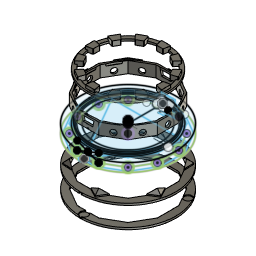
ARC4 v7 (Autodesk Fusion 360 design; units mm, degrees)
Autodesk Fusion 360 part; units mm, degrees
sketch "Sketch1" plane through (0, 0, 0) normal (0, 0, 1) x (1, 0, 0)
  circle A0 centre (0, 0) radius 40
  circle A1 centre (0, 0) radius 39
  circle A2 centre (0, 0) radius 34
  line L0 (0, 0) -> (0, 40)
  circle A3 centre (0, 36.5) radius 2.5
  circle A4 centre (0, 36.5) radius 3.5
  line L1 (3.5, 40) -> (-3.5, 40)
  line L2 (-3.5, 40) -> (-3.5, 33)
  line L3 (-3.5, 33) -> (3.0958, 33)
  line L4 (3.5, 33) -> (3.5, 40)
  line L5 (3.5, 40) -> (-3.5, 33) construction
  line L6 (-3.5, 40) -> (3.5, 33) construction
  line L7 (4.3815, 40) -> (-4.5, 40)
  line L8 (-5, 39.5) -> (-5, 33)
  line L9 (-3.0958, 33) -> (5, 33)
  line L10 (5, 33) -> (5, 40)
  line L11 (5, 40) -> (-5, 33) construction
  line L12 (-5, 40) -> (5, 33) construction
  line L13 (-5, 40) -> (-3.5847, 33.3952)
  line L14 (3.5847, 33.3952) -> (4.8704, 39.3952)
  arc A5 (-4.5, 40) -> (-5, 39.5) centre (-4.5, 39.5) ccw
  arc A6 (4.8704, 39.3952) -> (4.3815, 40) centre (4.3815, 39.5) ccw
  arc A7 (-3.5847, 33.3952) -> (-3.0958, 33) centre (-3.0958, 33.5) ccw
  arc A8 (3.0958, 33) -> (3.5847, 33.3952) centre (3.0958, 33.5) ccw
  line L15 (-10.718, 40) -> (-29.282, 29.282)
  line L16 (-29.282, 29.282) -> (-40, 10.718)
  line L17 (-40, 10.718) -> (-40, -10.718)
  line L18 (-40, -10.718) -> (-29.282, -29.282)
  line L19 (-29.282, -29.282) -> (-10.718, -40)
  line L20 (-10.718, -40) -> (10.718, -40)
  line L21 (10.718, -40) -> (29.282, -29.282)
  line L22 (29.282, -29.282) -> (40, -10.718)
  line L23 (40, -10.718) -> (40, 10.718)
  line L24 (40, 10.718) -> (29.282, 29.282)
  line L25 (29.282, 29.282) -> (10.718, 40)
  line L26 (10.718, 40) -> (-10.718, 40)
  circle A9 centre (0, 0) radius 38
  circle A10 centre (0, 0) radius 42
  line L27 (0, 0) -> (42, 0) construction
  line L28 (-11.2539, 42) -> (-30.7461, 30.7461)
  line L29 (-30.7461, 30.7461) -> (-42, 11.2539)
  line L30 (-42, 11.2539) -> (-42, -11.2539)
  line L31 (-42, -11.2539) -> (-30.7461, -30.7461)
  line L32 (-30.7461, -30.7461) -> (-11.2539, -42)
  line L33 (-11.2539, -42) -> (11.2539, -42)
  line L34 (11.2539, -42) -> (30.7461, -30.7461)
  line L35 (30.7461, -30.7461) -> (42, -11.2539)
  line L36 (42, -11.2539) -> (42, 11.2539)
  line L37 (42, 11.2539) -> (30.7461, 30.7461)
  line L38 (30.7461, 30.7461) -> (11.2539, 42)
  line L39 (11.2539, 42) -> (-11.2539, 42)
  circle A11 centre (0, 0) radius 50
  point P0 (0, 36.5)
  point P1 (0, 36.5)
  dimension "d1" = 80
  dimension "d2" = 78
  dimension "d3" = 68
  dimension "d4" = 7
  dimension "d5" = 7
  dimension "d6" = 10
  dimension "d7" = 7
  dimension "d8" = 0.5
  dimension "d9" = 0.5
  dimension "d19" = 76
  dimension "d20" = 84
  dimension "d37" = 100
  constraint coincident A0.centre A1.centre
  constraint concentric A0 A1
  constraint concentric A0 A2
  constraint coincident A0 L0.end
  constraint vertical L0
  constraint tangent A2 A3
  constraint concentric A3 A4
  constraint coincident L0.end A4
  constraint tangent A0 A4
  constraint horizontal L1
  constraint perpendicular L1 L2
  constraint parallel L1 L3
  constraint parallel L2 L4
  constraint coincident L5 P1
  constraint coincident L6 P1
  constraint coincident P1 P0
  constraint horizontal L7
  constraint perpendicular L7 L8
  constraint parallel L7 L9
  constraint parallel L8 L10
  constraint coincident L11 P1
  constraint coincident L12 P1
  constraint coincident L12.start L7
  constraint coincident L12.start L8
  constraint tangent L7 A5
  constraint tangent L8 A5
  constraint coincident L10.end L7
  constraint coincident L10.end L14
  constraint tangent L7 A6
  constraint tangent L14 A6
  constraint equal A5 A6
  constraint coincident L2.end L13
  constraint coincident L8.end L9
  constraint tangent L13 A7
  constraint tangent L9 A7
  constraint coincident L4.start L14
  constraint coincident L4.start L3
  constraint tangent L14 A8
  constraint tangent L3 A8
  constraint equal A7 A8
  constraint concentric A1 A9
  constraint horizontal L27
  constraint concentric A1 A11
  measures "d1" diameter of A0
  measures "d2" diameter of A1
  measures "d3" diameter of A2
  measures "d4" distance of L2.end L4.start
  measures "d5" distance of L1.end L2.end
  measures "d6" distance of L8.end L9.end
  measures "d7" distance of L12.start L8.end
  measures "d8" radius of A5
  measures "d9" radius of A7
  measures "d19" diameter of A9
  measures "d20" diameter of A10
  measures "d37" diameter of A11
extrude "Extrude1" add sketch "Sketch1" along normal blind 2 contours A0 A1 L8 L10 A5 | A0 L22 L23 | A0 L23 L24 | A0 L24 L25 | A0 L21 L22 | A0 L10 L25 L26 | A0 L20 L21 | A0 A1 L10 L14 A6 | A0 L10 A6 L26 | A0 L19 L20 | A1 L10 L14 A9 | A1 L8 L10 A9 | A0 L18 L19 | A0 L17 L18 | A0 A1 L8 L13 A5 | A1 L8 L13 A9 | A0 L16 L17 | A0 L15 L16 | L13 A5 L26 | A0 L13 A5 L15 L26 | A10 makes body 1
extrude "Extrude2" add sketch "Sketch1" along normal blind 5 separate body contours A0 A1 L4 L14 A6 | A0 L4 L7 A6 L26 | A0 A1 A4 L4 | A0 L1 L4 L7 L26 | A1 L4 L14 A9 | A0 A1 A4 L2 | A1 L0 A4 | A1 L0 A4 | A0 L1 L2 L7 L26 | A1 A4 L4 A9 | A2 L4 L14 A9 | A0 A1 L2 L13 | A0 L2 L7 L13 A5 L26 | A1 A3 A4 A9 | L0 A3 A9 | A1 A3 A4 A9 | L0 A3 A9 | A1 A4 L2 A9 | A4 L4 A9 | A1 L2 L13 A9 | A2 L4 L14 A8 | A0 L13 A5 | L0 A3 A9 | L0 A3 A9 | A2 A3 A4 A9 | A2 A3 A4 A9 | A4 L2 A9 | A2 A4 L4 | A2 L2 L13 A9 | A2 A4 L3 L4 L9 A8 | A2 L0 A4 | A2 L0 A4 | A2 A4 L2 | A2 L2 L13 A7 | A2 A4 L2 L3 L9 A7 makes body 2
pattern_circular "C-Pattern1" count 12 over 360 about axis through (0, 0, 1.75) along (0, 0, 1) of bodies 2 makes body 3 at (-17.1521, 32.7176, 0) makes body 4 at (-31.213, 19.7582, 0) makes body 5 at (-36.9103, 1.5046, 0) makes body 6 at (-32.7176, -17.1521, 0) makes body 7 at (-19.7582, -31.213, 0) makes body 8 at (-1.5046, -36.9103, 0) makes body 9 at (17.1521, -32.7176, 0) makes body 10 at (31.213, -19.7582, 0) makes body 11 at (36.9103, -1.5046, 0) makes body 12 at (32.7176, 17.1521, 0) makes body 13 at (19.7582, 31.213, 0)
combine "Combine1" operation add target body 4 tool bodies 9 2 10 8 13 12 1 11 7 6 3 5
hole "Hole1" at (0, 36.5, 0) direction (0, 0, 1) diameter 3.5 depth 3 tip angle 140 bodies 4
pattern_circular "C-Pattern2" count 12 over 360 about axis through (0, 0, 1.75) along (0, 0, 1) of "Hole1"
extrude "Extrude3" add sketch "Sketch1" against normal blind 9 separate body contours A10 | A10 L35 L36 | A10 L36 L37 | A10 L37 L38 | A10 L34 L35 | A10 L38 L39 | A10 L33 L34 | A10 L28 L39 | A10 L32 L33 | A10 L28 L29 | A10 L31 L32 | A10 L29 L30 | A10 L30 L31 makes body 14
extrude "Extrude4" add sketch "Sketch1" along normal blind 2 from surface at -9 separate body contours A11 makes body 15
sketch "Sketch2" plane through (0, -42, 0) normal (0, -1, 0) x (1, 0, 0)
  line L0 (11.2539, 0) -> (-11.2539, 0)
  line L1 (-11.2539, 0) -> (-11.2539, -9)
  line L2 (-11.2539, -9) -> (11.2539, -9)
  line L3 (11.2539, -9) -> (11.2539, 0)
  line L4 (-11.2539, 0) -> (11.2539, -9)
  line L5 (-11.2539, -9) -> (11.2539, 0)
  circle A0 centre (0, -4.5) radius 2.9
  dimension "d31" = 5.8
  constraint coincident L0.end L1.start
  constraint coincident L2.end L3.start
  constraint coincident L1.end L2.start
  constraint coincident L0.start L3.end
  constraint midpoint L5 A0.centre
  measures "d31" diameter of A0
hole "Hole2" at (0, -42, -4.5) direction (0, 1, 0) diameter 5.8 depth 10 tip angle 140 bodies 14
pattern_circular "C-Pattern3" count 12 over 360 about axis through (0, 0, 1.75) along (0, 0, 1) of "Hole2"
sketch "Sketch4" plane through (0, 0, -9) normal (0, 0, 1) x (1, 0, 0)
  line L0 (-11.2539, 42) -> (11.2539, 42)
  line L1 (-30.7461, 30.7461) -> (-11.2539, 42)
  line L2 (-42, 11.2539) -> (-30.7461, 30.7461)
  line L3 (-42, -11.2539) -> (-42, 11.2539)
  line L4 (-30.7461, -30.7461) -> (-42, -11.2539)
  line L5 (-11.2539, -42) -> (-30.7461, -30.7461)
  line L6 (11.2539, -42) -> (-11.2539, -42)
  line L7 (30.7461, -30.7461) -> (11.2539, -42)
  line L8 (42, -11.2539) -> (30.7461, -30.7461)
  line L9 (42, 11.2539) -> (42, -11.2539)
  line L10 (30.7461, 30.7461) -> (42, 11.2539)
  circle A0 centre (0, 0) radius 50
  line L11 (0, -46) -> (39.8372, 23)
  line L12 (39.8372, 23) -> (-39.8372, 23)
  line L13 (-39.8372, 23) -> (0, -46)
  circle A1 centre (0, -46) radius 4.1
  line L14 (30.7461, 30.7461) -> (11.2539, 42)
  line L15 (11.2539, 42) -> (-11.2539, 42)
  line L16 (-11.2539, 42) -> (-30.7461, 30.7461)
  line L17 (-30.7461, 30.7461) -> (-42, 11.2539)
  line L18 (-42, 11.2539) -> (-42, -11.2539)
  line L19 (-42, -11.2539) -> (-30.7461, -30.7461)
  line L20 (-30.7461, -30.7461) -> (-11.2539, -42)
  line L21 (-11.2539, -42) -> (11.2539, -42)
  line L22 (11.2539, -42) -> (30.7461, -30.7461)
  line L23 (30.7461, -30.7461) -> (42, -11.2539)
  line L24 (42, -11.2539) -> (42, 11.2539)
  line L25 (42, 11.2539) -> (30.7461, 30.7461)
  circle A2 centre (0, 0) radius 50
  line L26 (11.2539, 42) -> (-11.2539, 42)
  line L27 (11.2539, 42) -> (0, 42)
  line L28 (3, 49.1142) -> (-3, 49.1142)
  line L29 (-3, 49.1142) -> (-3, 34.8858)
  line L30 (-3, 34.8858) -> (3, 34.8858)
  line L31 (3, 34.8858) -> (3, 49.1142)
  line L32 (3, 49.1142) -> (-3, 34.8858) construction
  line L33 (-3, 49.1142) -> (3, 34.8858) construction
  line L34 (-12.5936, 47) -> (-34.4064, 34.4064)
  line L35 (-34.4064, 34.4064) -> (-47, 12.5936)
  line L36 (-47, 12.5936) -> (-47, -12.5936)
  line L37 (-47, -12.5936) -> (-34.4064, -34.4064)
  line L38 (-34.4064, -34.4064) -> (-12.5936, -47)
  line L39 (-12.5936, -47) -> (12.5936, -47)
  line L40 (12.5936, -47) -> (34.4064, -34.4064)
  line L41 (34.4064, -34.4064) -> (47, -12.5936)
  line L42 (47, -12.5936) -> (47, 12.5936)
  line L43 (47, 12.5936) -> (34.4064, 34.4064)
  line L44 (34.4064, 34.4064) -> (12.5936, 47)
  line L45 (12.5936, 47) -> (-12.5936, 47)
  line L46 (11.2539, 42) -> (12.5936, 47)
  line L47 (12.5936, 47) -> (3, 42)
  line L48 (12.5936, 47) -> (18.4019, 37.8731)
  line L49 (0, 42) -> (0, 49.1142)
  line L50 (-12.5936, 47) -> (-3, 42)
  line L51 (-12.5936, 47) -> (-18.4019, 37.8731)
  point P0 (0, 42)
  dimension "d38" = 8.2
  dimension "d48" = 6
  dimension "d49" = 47
  constraint coincident A0.centre A2.centre
  constraint coincident L11.start L13.end
  constraint coincident L0.end L14.end
  constraint coincident L0.start L1.end
  constraint midpoint L26 P0
  constraint horizontal L28
  constraint perpendicular L28 L29
  constraint parallel L28 L30
  constraint parallel L29 L31
  constraint coincident L32 P0
  constraint coincident L33 P0
  constraint coincident P0 L27.end
  constraint midpoint L31 L47.end
  constraint symmetric L44.end L46 L45.start
  constraint symmetric L46 L47.end L48.end
  constraint midpoint L28 L49.end
  constraint symmetric L44.end L49 L34.start
  constraint symmetric L47.end L49 L50.end
  constraint symmetric L48.end L49 L51.end
  measures "d38" diameter of A1
  measures "d48" distance of L29.end L30.end
  measures "d49" distance of A0.centre L45
hole "Hole3" at (0, -46, -9) direction (0, 0, 1) diameter 8.2 depth 1 tip angle 180 bodies 14 15
pattern_circular "C-Pattern4" count 3 over 360 about axis through (0, 0, 1.75) along (0, 0, 1) of "Hole3"
extrude "Extrude5" add sketch "Sketch1" along normal blind 4 separate body contours A10 L36 L37 | A10 L34 L35 | A10 L38 L39 | A10 L32 L33 | A10 L28 L29 | A10 L30 L31 makes body 16 at (38.0649, 17.75, 2.6667) makes body 17 at (-37.2545, -19.3934, 2.6667) makes body 18 at (35.4224, -22.5666, 2.6667) makes body 19 at (19.3934, 37.2545, 1.3333) makes body 20 at (-35.4224, 22.5666, 2.6667) makes body 21 at (-3.6605, -41.8402, 1.3333)
combine "Combine2" operation add target body 14 tool bodies 16 17 18 19 20 21
extrude "Extrude6" add sketch "Sketch4" along normal blind 7 separate body contours L0 L1 L15 L16 L26 L50 L51 makes body 22
chamfer "Chamfer1" distance 3.8 angle 45 2 edges at (-7.7968, 44.5, -2) (-15.4978, 42.4365, -2) on bodies 22
pattern_circular "C-Pattern5" count 6 over 360 about axis through (0, 0, 1.75) along (0, 0, 1) of bodies 22 makes body 23 at (-42, 8.4919, -5.6) makes body 24 at (-32.1271, -28.3542, -5.6) makes body 25 at (8.4919, -42, -5.6) makes body 26 at (42, -8.4919, -5.6) makes body 27 at (28.3542, 32.1271, -5.6)
combine "Combine3" operation add target body 27 tool bodies 26 25 24 23 22 15
extrude "Extrude7" add 1 faces at (-20.3333, 35.2184, 0) along direction (0, 0, 1) blind 3 on bodies 14 bodies 14
sketch "Sketch5" plane through (0, 0, 3) normal (0, 0, 1) x (-1, 0, 0)
  arc A0 (21, 36.3731) -> (0, 42) centre (0, 0) ccw
  line L0 (0, 42) -> (-11.2539, 42)
  line L1 (-11.2539, 42) -> (-21, 36.3731)
  arc A1 (-21, 36.3731) -> (-36.3731, 21) centre (0, 0) ccw
  line L2 (-36.3731, 21) -> (-42, 11.2539)
  line L3 (-42, 11.2539) -> (-42, 0)
  arc A2 (-42, 0) -> (-36.3731, -21) centre (0, 0) ccw
  line L4 (-36.3731, -21) -> (-30.7461, -30.7461)
  line L5 (-30.7461, -30.7461) -> (-21, -36.3731)
  arc A3 (-21, -36.3731) -> (0, -42) centre (0, 0) ccw
  line L6 (0, -42) -> (11.2539, -42)
  line L7 (11.2539, -42) -> (21, -36.3731)
  arc A4 (21, -36.3731) -> (36.3731, -21) centre (0, 0) ccw
  line L8 (36.3731, -21) -> (42, -11.2539)
  line L9 (42, -11.2539) -> (42, 0)
  arc A5 (42, 0) -> (36.3731, 21) centre (0, 0) ccw
  line L10 (36.3731, 21) -> (30.7461, 30.7461)
  line L11 (30.7461, 30.7461) -> (21, 36.3731)
  line L12 (10.718, -40) -> (-10.718, -40)
  line L13 (-10.718, -40) -> (-29.282, -29.282)
  line L14 (-29.282, -29.282) -> (-40, -10.718)
  line L15 (-40, -10.718) -> (-40, 10.718)
  line L16 (-40, 10.718) -> (-29.282, 29.282)
  line L17 (-29.282, 29.282) -> (-10.718, 40)
  line L18 (-10.718, 40) -> (10.718, 40)
  line L19 (10.718, 40) -> (29.282, 29.282)
  line L20 (29.282, 29.282) -> (40, 10.718)
  line L21 (40, 10.718) -> (40, -10.718)
  line L22 (40, -10.718) -> (29.282, -29.282)
  line L23 (29.282, -29.282) -> (10.718, -40)
  circle A6 centre (0, 0) radius 40.5
  dimension "d57" = 81
  constraint coincident A0.centre A1.centre
  measures "d57" diameter of A6
extrude "Extrude8" cut sketch "Sketch5" against normal blind 2 contours L12 A6 | L12 L13 L14 L15 L16 L17 L18 L19 L20 L21 L22 L23 A6 | L22 A6 | L14 A6 | L21 A6 | L15 A6 | L20 A6 | L16 A6 | L19 A6 | L17 A6 | L18 A6 bodies 14
move_body "Move1" bodies 4 to x (1, 0, 0) y (0, 1, 0) z (0, 0, 1) at (0, 0, 3)
extrude "Extrude9" add sketch "Sketch4" against normal blind 2 separate body contours L0 L1 L15 L16 L26 L50 L51 | L0 L15 L26 L29 L45 L49 | L29 L45 L50 | L1 L2 L3 L4 L5 L6 L12 L13 A1 L16 L17 L18 L19 L20 L21 L34 L35 L36 L37 L38 L39 L51 | L0 L15 L26 L27 L31 L45 L49 | A0 A1 A2 L28 L29 L31 L34 L35 L36 L37 L38 L39 L40 L41 L42 L43 L44 L45 | L28 L29 L45 L49 | L0 L15 L26 L27 L46 L47 | L31 L45 L47 | L28 L31 L45 L49 | L2 L12 L13 L17 | L14 L46 L48 | L6 L7 L8 L9 L10 L11 L12 A1 L14 L21 L22 L23 L24 L25 L39 L40 L41 L42 L43 L44 L48 | L10 L11 L12 L25 | L6 L11 L13 A1 L21 | L11 L13 A1 L39 | A0 A1 A2 L39 makes body 28
hole "Hole4" at (0, -46, -9) at (-39.8372, 23, -9) at (39.8372, 23, -9) direction (0, 0, -1) diameter 8.2 depth 1 tip angle 180 bodies 28
sketch "Sketch6" plane through (0, 42, 0) normal (0, 1, 0) x (-1, 0, 0)
  circle A0 centre (0, -4.5) radius 2.9
  line L0 (-11.2539, 4) -> (-11.2539, -9)
  line L1 (-11.2539, -9) -> (11.2539, -9)
  line L2 (11.2539, -9) -> (11.2539, 3)
  line L3 (11.2539, 3) -> (0, 3)
  line L4 (0, 3) -> (0, 4)
  line L5 (0, 4) -> (-11.2539, 4)
  line L6 (7, 4) -> (-7, 4)
  line L7 (-7, 4) -> (-7, -13)
  line L8 (-7, -13) -> (7, -13)
  line L9 (7, -13) -> (7, 4)
  line L10 (7, 4) -> (-7, -13) construction
  line L11 (-7, 4) -> (7, -13) construction
  line L12 (5, 4) -> (-5, 4)
  line L13 (-5, 4) -> (-5, -13)
  line L14 (-5, -13) -> (5, -13)
  line L15 (5, -13) -> (5, 4)
  line L16 (5, 4) -> (-5, -13) construction
  line L17 (-5, 4) -> (5, -13) construction
  line L18 (-5, -4.5) -> (7, -4.5)
  line L19 (-7, 4) -> (-5, -4.5)
  line L20 (7, 4) -> (5, -4.5)
  line L21 (-7, 1) -> (7, 1)
  point P0 (0, -4.5)
  point P1 (0, -4.5)
  constraint horizontal L6
  constraint perpendicular L6 L7
  constraint parallel L6 L8
  constraint parallel L7 L9
  constraint coincident L10 P1
  constraint coincident L11 P1
  constraint coincident P0 A0.centre
  constraint horizontal L12
  constraint perpendicular L12 L13
  constraint parallel L12 L14
  constraint parallel L13 L15
  constraint coincident L16 P1
  constraint coincident L17 P1
  constraint coincident L6 L12.start
  constraint coincident P1 P0
  constraint midpoint L13 L18.start
  constraint midpoint L9 L18.end
  constraint midpoint L15 L20.end
  constraint coincident L7 L21.start
  constraint coincident L9 L21.end
  constraint perpendicular L9 L21
extrude "Extrude10" cut sketch "Sketch6" against normal blind 93 contours A0 L13 L15 L18 L21 | L15 L20 L21 | L13 L19 L21 bodies 14
extrude "Extrude11" add sketch "Sketch6" against normal blind 2 contours A0 L18 picked at (-0.0722, -5.464) bodies 14
extrude "Extrude12" add sketch "Sketch6" against normal blind 2 from surface at -82 contours A0 L18 picked at (-0.0722, -5.464) bodies 14
move_body "Move2" bodies 4 to x (1, 0, 0) y (0, 1, 0) z (0, 0, 1) at (0, 0, 45)
move_body "Move3" bodies 14 to x (1, 0, 0) y (0, 1, 0) z (0, 0, 1) at (0, 0, 25)
move_body "Move4" bodies 28 to x (1, 0, 0) y (0, 1, 0) z (0, 0, 1) at (0, 0, -50)
move_body "Move5" bodies 27 to x (1, 0, 0) y (0, 1, 0) z (0, 0, 1) at (0, 0, -30)
